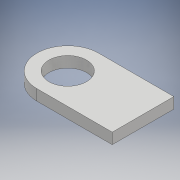
# Autodesk Inventor part: tipper_link_D_spacer
Saved by Autodesk Inventor 2017 (Build 210142000, 142)
## iProperties
Created: 2017-07-15
Part Number: tipper_link_D_spacer
Material: Generic
Document SubType Name: Modeling
Designer: Nic
Density: 1 g/cm^3
Appearance: Default
Author: Nic
Autodesk Inventor part; units mm, degrees
ref_plane "YZ Plane" through (0, 0, 0) normal (1, 0, 0) x (0, 1, 0)
ref_plane "XZ Plane" through (0, 0, 0) normal (0, 1, 0) x (-1, 0, 0)
ref_plane "XY Plane" through (0, 0, 0) normal (0, 0, 1) x (1, 0, 0)
sketch "Sketch1" plane through (0, 0, 0) normal (0, 0, 1) x (1, 0, 0)
  circle A0 centre (0, 0) radius 5.5
  line L0 (0, 9) -> (22, 9)
  line L1 (22, -9) -> (0, -9)
  arc A1 (0, 9) -> (0, -9) centre (0, 0) ccw
  line L2 (22, 9) -> (22, -9)
  dimension "d0" = 11
  dimension "d1" = 9
  dimension "d9" = 22
  constraints: 6 end point, 2 centre point, 2 point on circle, 2 tangent, 1 coincident, 1 concentric, 1 horizontal, 1 parallel, 1 vertical
  measures "d0" diameter of A0
  measures "d1" radius of A1
  measures "d9" distance from line of point (0, 0) L2
extrude "Extrusion1" add sketch "Sketch1" along normal blind 3.175
body "Solid1"
